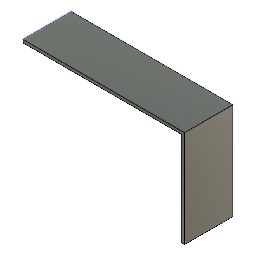
sort_bin (Autodesk Fusion 360 design; units mm, degrees)
Autodesk Fusion 360 part; units mm, degrees
sketch "Sketch1" plane through (0, 0, 0) normal (0, 0, 1) x (1, 0, 0)
  line L0 (0, 0) -> (40, 0)
  line L1 (40, 0) -> (40, 30)
  line L2 (40, 30) -> (0, 30)
  line L3 (0, 30) -> (0, 0)
  dimension "d1" = 40
  dimension "d2" = 30
  constraint horizontal L0
  constraint vertical L1
  constraint horizontal L2
  constraint vertical L3
  constraint coincident L0.start L3.end
  measures "d1" distance of L0.start L0.end
  measures "d2" distance of L0.start L2.end
extrude "Extrude1" add sketch "Sketch1" along normal blind 2
sketch "Sketch2" plane through (0, 0, 2) normal (0, 0, 1) x (-1, 0, 0)
  line L0 (0, -30) -> (0, 0)
  line L1 (0, 0) -> (-40, 0)
  line L2 (-40, 0) -> (-40, -30)
  line L3 (-40, -30) -> (0, -30)
  line L4 (-9, -30) -> (-10, -30)
  line L5 (-10, -30) -> (-10, 0)
  line L6 (-10, 0) -> (-9, 0)
  line L7 (-9, 0) -> (-9, -30)
  dimension "d5" = 1
  dimension "d6" = 30
  dimension "d7" = 9
  constraint horizontal L4
  constraint vertical L5
  constraint horizontal L6
  constraint vertical L7
  constraint coincident L3 L4.start
  measures "d5" distance of L4.start L4.end
  measures "d6" distance of L4.start L6.end
  measures "d7" distance of L0 L7
extrude "Extrude2" cut sketch "Sketch2" against normal blind 1 contours L1 L3 L4 L5 L6 L7
sketch "Sketch4" plane through (0, 0, 0) normal (0, 0, -1) x (1, 0, 0)
  line L0 (0, 0) -> (0, -30)
  line L1 (0, -30) -> (40, -30)
  line L2 (40, -30) -> (40, 0)
  line L3 (40, 0) -> (0, 0)
  line L4 (40, 0) -> (38, 0)
  line L5 (38, 0) -> (38, -30)
  line L6 (38, -30) -> (40, -30)
  line L7 (40, -30) -> (40, 0)
  constraint horizontal L4
  constraint vertical L5
  constraint horizontal L6
  constraint vertical L7
  constraint coincident L1 L5.end
  constraint coincident L2.end L3.start
extrude "Extrude3" add sketch "Sketch4" along normal blind 58 contours L1 L2 L3 L4 L5 L6 L7
extrude "Extrude4" add 1 faces at (0, 20, 0.6667) along direction (-1, 0, 0) blind 60
extrude "Extrude5" add 1 faces at (9.3333, 20, 1) along direction (0, 0, 1) blind 1
sketch "Sketch5" plane through (0, 0, 2) normal (0, 0, 1) x (-1, 0, 0)
  line L0 (-40, -30) -> (60, -30)
  line L1 (60, -30) -> (60, 0)
  line L2 (60, 0) -> (-40, 0)
  line L3 (-40, 0) -> (-40, -30)
  line L4 (11, 0) -> (10, 0)
  line L5 (10, 0) -> (10, -30)
  line L6 (10, -30) -> (11, -30)
  line L7 (11, -30) -> (11, 0)
  dimension "d18" = 1
  dimension "d19" = 30
  dimension "d20" = 49
  constraint horizontal L4
  constraint vertical L5
  constraint horizontal L6
  constraint vertical L7
  constraint coincident L2 L4.start
  measures "d18" distance of L4.start L4.end
  measures "d19" distance of L4.start L6.end
  measures "d20" distance of L1 L7
extrude "Extrude6" cut sketch "Sketch5" along normal blind 1 contours L0 L2 L4 L5 L6 L7
sketch "Sketch6" plane through (0, 0, 2) normal (0, 0, 1) x (-1, 0, 0)
  line L0 (60, 0) -> (-40, 0)
  line L1 (-40, 0) -> (-40, -30)
  line L2 (-40, -30) -> (60, -30)
  line L3 (60, -30) -> (60, 0)
equation "d21 = mm"
